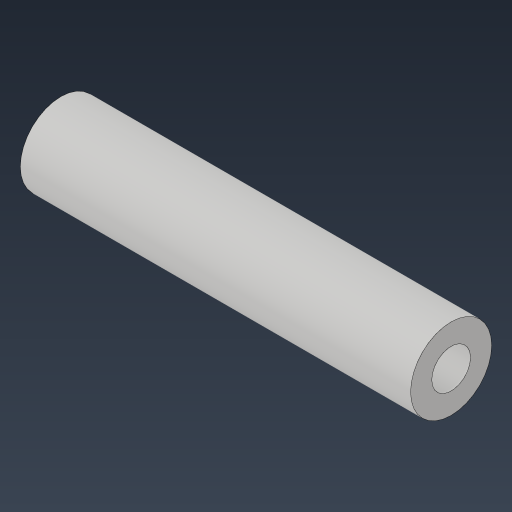
# Autodesk Inventor part: Dribblerschnecke v4
Saved by Autodesk Inventor 2023.1 (Build 271208000, 208)
## iProperties
Part Number: Dribblerschnecke v4
Material: Generisch
Document SubType Name: Modeling
Designer: rYan
Density: 1 g/cm^3
Appearance: Vorgabe
Author: rYan
Autodesk Inventor part; units mm, degrees
ref_plane "YZ Plane" through (0, 0, 0) normal (1, 0, 0) x (0, 1, 0)
ref_plane "XZ Plane" through (0, 0, 0) normal (0, 1, 0) x (-1, 0, 0)
ref_plane "XY Plane" through (0, 0, 0) normal (0, 0, 1) x (1, 0, 0)
sketch "Skizze1" plane through (0, 0, 0) normal (1, 0, 0) x (0, 1, 0)
  circle A0 centre (0, 0) radius 3.35
  circle A1 centre (0, 0) radius 5.5
  dimension "d0" = 6.7
  dimension "d1" = 11
  constraints: 2 centre point, 2 coincident
  measures "d0" diameter of A0
  measures "d1" diameter of A1
extrude "Extrusion1" add sketch "Skizze1" along normal mid plane 67.4
sketch "Skizze2" plane through (0, 0, 0) normal (0, 1, 0) x (-1, 0, 0)
  line L0 (33.7, 5.5) -> (33.7, 3.35) projected
  line L1 (33.7, 3.35) -> (-33.7, 3.35) projected
  line L2 (-33.7, 3.35) -> (-33.7, 5.5) projected
  line L3 (-33.7, 5.5) -> (33.7, 5.5) projected
  line L4 (33.7, -3.35) -> (33.7, -5.5) projected
  line L5 (33.7, -5.5) -> (-33.7, -5.5) projected
  line L6 (-33.7, -5.5) -> (-33.7, -3.35) projected
  line L7 (-33.7, -3.35) -> (33.7, -3.35) projected
  line L8 (-50.7835, 0) -> (68.8013, 0) projected
  line L9 (33.7, 5.5) -> (25.7, 7)
  line L10 (25.7, 7) -> (25.7, 5.5)
  circle A0 centre (30.2177, 28.0276) radius 21.5 construction
  line L11 (30.2177, 28.0276) -> (30.2177, 6.5276) construction
  line L12 (33.7, 5.5) -> (34.7, 5.5) construction
  line L13 (34.7, 5.5) -> (34.7, 7) construction
  line L14 (34.7, 7) -> (42.7, 5.5) construction
  line L15 (42.7, 5.5) -> (34.7, 5.5) construction
  line L16 (34.7, 7) -> (25.7, 7) construction
  line L17 (25.7, 7) -> (24.2, 5.5)
  point P0 (0, 0)
  dimension "d4" = 43
  dimension "d6" = 1.5
  dimension "d16" = 8
  dimension "d17" = 8
  dimension "d18" = 9
  dimension "d20" = 45
  constraints: 18 end point, 4 point on line, 2 perpendicular, 2 point on circle, 1 centre point, 1 collinear, 1 horizontal, 1 tangent, 1 vertical
  measures "d4" diameter of A0
  measures "d6" distance of L9.end L10.end
  measures "d16" distance between parallel lines of L0 L10
  measures "d17" distance from line of L14.end L13
  measures "d18" distance between parallel lines of L10 L13
  measures "d20" angle of L10 L17
feature "Spirale1" [suppressed]
mirror "Spiegeln1" [suppressed]
sketch "Skizze4" plane through (33.7, 0, 0) normal (1, 0, 0) x (0, 0, -1)
  circle A0 centre (0, 0) radius 6
  circle A1 centre (0, 0) radius 5.5 projected
  point P0 (0, 5.5)
  dimension "d21" = 12
  constraints: 1 centre point, 1 coincident, 1 vertical alignment
  measures "d21" diameter of A0
extrude "Extrusion2" [suppressed]
sketch "Skizze5" plane through (0, 0, 0) normal (0, 1, 0) x (-1, 0, 0)
  line L0 (33.7, 3.35) -> (-33.7, 3.35) projected
  line L1 (-33.7, -3.35) -> (33.7, -3.35) projected
  circle A0 centre (21.2, 28.0581) radius 21.5
  line L2 (33.7, 5.5) -> (33.7, 3.35) projected
  line L3 (-33.7, 3.35) -> (-33.7, 5.5) projected
  line L4 (-33.7, 5.5) -> (33.7, 5.5) projected
  line L5 (33.7, -3.35) -> (33.7, -5.5) projected
  line L6 (33.7, -5.5) -> (-33.7, -5.5) projected
  line L7 (-33.7, -5.5) -> (-33.7, -3.35) projected
  point P0 (0, 0)
  dimension "d25" = 43
  constraints: 1 centre point
  measures "d25" diameter of A0
sketch "Skizze6" plane through (-33.7, 0, 0) normal (-1, 0, 0) x (0, 0, 1)
  circle A0 centre (0, 0) radius 5.5 projected
  circle A1 centre (0, 0) radius 7
  dimension "d26" = 14
  constraints: 1 centre point, 1 coincident
  measures "d26" diameter of A1
extrude "Extrusion3" add sketch "Skizze6" against normal up to surface (67.4 mm away)
equation "\"d17\" = d16"
